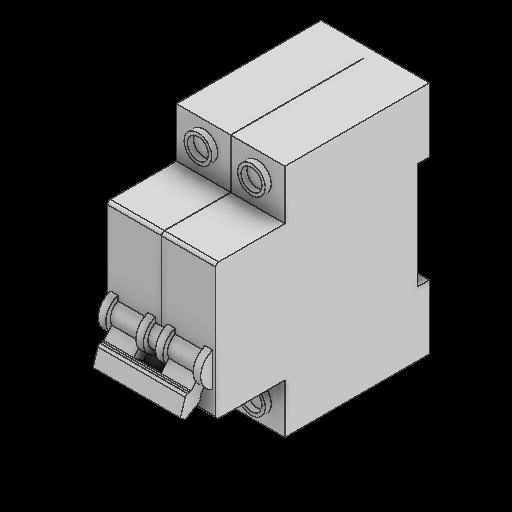
# Autodesk Inventor part: Breaker
Saved by Autodesk Inventor 2025.2 (Build 292293000, 293)
## iProperties
Created: 2026-05-14
Part Number: Breaker
Material: Generic
Document SubType Name: Modeling
Designer: valer
Density: 1 g/cm^3
Appearance: Default
Author: valer
Autodesk Inventor part; units mm, degrees
ref_plane "YZ Plane" through (0, 0, 0) normal (1, 0, 0) x (0, 1, 0)
ref_plane "XZ Plane" through (0, 0, 0) normal (0, 1, 0) x (-1, 0, 0)
ref_plane "XY Plane" through (0, 0, 0) normal (0, 0, 1) x (1, 0, 0)
sketch "Base" plane through (0, 0, 0) normal (0, 0, 1) x (1, 0, 0)
  line L0 (-18, -39) -> (18, -39)
  line L1 (18, -39) -> (18, 39)
  line L2 (18, 39) -> (-18, 39)
  line L3 (-18, 39) -> (-18, -39)
  line L4 (-18, -39) -> (18, 39) construction
  line L5 (18, -39) -> (-18, 39) construction
  point P0 (0, 0)
  dimension "d0" = 78
  dimension "d1" = 36
  constraints: 12 end point, 2 midpoint, 2 parallel, 1 horizontal, 1 perpendicular
  measures "d0" distance of L2.end L0.start
  measures "d1" distance of L0.start L0.end
extrude "BaseFeature" add sketch "Base" along normal blind 48
sketch "DINRail" plane through (-18, -39, 0) normal (-1, 0, 0) x (0, 0, 1)
  line L0 (0, 78) -> (0, 0) construction
  line L1 (0, 0) -> (48, 0) construction
  line L2 (48, 78) -> (48, 0) construction
  line L3 (0, 78) -> (48, 78) construction
  line L4 (0, 56.7) -> (4, 56.7)
  line L5 (4, 56.7) -> (4, 21.3)
  line L6 (4, 21.3) -> (0, 21.3)
  line L7 (0, 21.3) -> (0, 56.7)
  line L8 (0, 56.7) -> (4, 21.3) construction
  line L9 (4, 56.7) -> (0, 21.3) construction
  line L10 (0, -15.6) -> (0, 93.6) projected
  line L11 (-9.6, 39) -> (57.6, 39) construction
  line L12 (0, 78) -> (0, 0) projected
  point P0 (2, 39)
  dimension "d4" = 4
  dimension "d5" = 35.4
  constraints: 12 end point, 2 midpoint, 2 parallel, 1 horizontal, 1 perpendicular, 1 point on line, 1 vertical, 2 other
  measures "d4" distance of L4.start L4.end
  measures "d5" distance of L6.end L4.start
extrude "DinRailFeature" cut sketch "DINRail" against normal through all
sketch "Top" plane through (0, 0, 48) normal (0, 0, 1) x (1, 0, 0)
  line L0 (18, -39) -> (18, 39) projected
  line L1 (-18, -22.5) -> (18, -22.5)
  line L2 (18, -22.5) -> (18, 22.5)
  line L3 (18, 22.5) -> (-18, 22.5)
  line L4 (-18, 22.5) -> (-18, -22.5)
  line L5 (-18, -22.5) -> (18, 22.5) construction
  line L6 (18, -22.5) -> (-18, 22.5) construction
  point P0 (0, 0)
  point P1 (18, -22.5)
  dimension "d31" = 45
  constraints: 12 end point, 2 midpoint, 2 parallel, 1 horizontal, 1 perpendicular, 1 point on line
  measures "d31" distance between parallel lines of L1 L3
extrude "TopFeature" add sketch "Top" along normal blind 23
fillet "TopFilletsFeature" radius 1 2 edges at (0, 22.5, 71) (0, -22.5, 71)
sketch "Sketch17" plane through (0, 0, 71) normal (0, 0, 1) x (1, 0, 0)
  line L0 (18, 39) -> (-18, 39) projected
  line L1 (-18, -39) -> (18, -39) projected
  line L2 (-0.05, 39) -> (0.05, 39)
  line L3 (0.05, 39) -> (0.05, -39)
  line L4 (0.05, -39) -> (-0.05, -39)
  line L5 (-0.05, -39) -> (-0.05, 39)
  line L6 (0, -54.6) -> (0, 54.6) construction
  point P0 (0, 0)
  point P1 (0, 39)
  dimension "d71" = 0.1
  constraints: 8 end point, 3 point on line, 2 parallel, 1 horizontal, 1 midpoint, 1 perpendicular
  measures "d71" distance between parallel lines of L3 L5
sketch "SwitchHood" plane through (18, -39, 48) normal (1, 0, 0) x (0, 0, -1)
  line L0 (-23, 60.5) -> (-23, 17.5) projected
  circle A0 centre (-21, 30.5) radius 6
  line L1 (-21, 30.5) -> (-27, 30.5) construction
  line L2 (-21, 30.5) -> (-21, 24.5) construction
  line L3 (0, 16.5) -> (-22, 16.5) projected
  point P0 (48, 39)
  point P1 (-23, 24.8431)
  point P2 (-23, 36.1569)
  dimension "d35" = 12
  dimension "d36" = 4
  dimension "d37" = 8
  constraints: 4 end point, 2 point on circle, 1 centre point, 1 horizontal, 1 vertical
  measures "d35" diameter of A0
  measures "d36" distance from line of L0 L1.end
  measures "d37" distance from line of L2.end L3
extrude "SwitchHoodFeature" add sketch "SwitchHood" against normal up to surface (36 mm away) contours L0 A0 picked at (-25.1519, 30.9874)
sketch "SwithCuts" plane through (0, 0, 71) normal (0, 0, 1) x (1, 0, 0)
  line L0 (18, -2.8431) -> (18, 21.5) projected
  line L1 (18, -14.1569) -> (-18, -14.1569) projected
  line L2 (18, -2.8431) -> (17, -2.8431)
  line L3 (17, -2.8431) -> (17, -14.1569)
  line L4 (17, -14.1569) -> (18, -14.1569)
  line L5 (18, -14.1569) -> (18, -2.8431)
  line L6 (0, 54.6) -> (0, -54.6) construction
  line L7 (-18, -2.8431) -> (-17, -2.8431)
  line L8 (-17, -2.8431) -> (-17, -14.1569)
  line L9 (-17, -14.1569) -> (-18, -14.1569)
  line L10 (-18, -14.1569) -> (-18, -2.8431)
  line L11 (-18, -2.8431) -> (18, -2.8431) projected
  line L12 (-2, -2.8431) -> (2, -2.8431)
  line L13 (2, -2.8431) -> (2, -14.1569)
  line L14 (2, -14.1569) -> (-2, -14.1569)
  line L15 (-2, -14.1569) -> (-2, -2.8431)
  line L16 (-17, -2.8431) -> (-2, -14.1569) construction
  line L17 (2, -2.8431) -> (17, -14.1569) construction
  line L18 (-14.5, -14.1569) -> (-4.5, -14.1569)
  line L19 (-4.5, -14.1569) -> (-4.5, -2.8431)
  line L20 (-4.5, -2.8431) -> (-14.5, -2.8431)
  line L21 (-14.5, -2.8431) -> (-14.5, -14.1569)
  line L22 (-14.5, -14.1569) -> (-4.5, -2.8431) construction
  line L23 (-4.5, -14.1569) -> (-14.5, -2.8431) construction
  line L24 (14.5, -14.1569) -> (4.5, -14.1569)
  line L25 (4.5, -14.1569) -> (4.5, -2.8431)
  line L26 (4.5, -2.8431) -> (14.5, -2.8431)
  line L27 (14.5, -2.8431) -> (14.5, -14.1569)
  point P0 (0, 0)
  point P1 (-9.5, -8.5)
  point P2 (14.5, -14.1569)
  point P3 (-4.5, -14.1569)
  point P4 (-4.5, -2.8431)
  point P5 (2, -2.8431)
  dimension "d40" = 1
  dimension "d41" = 2
  dimension "d42" = 2
  dimension "d43" = 10
  constraints: 48 end point, 8 symmetric about line, 6 parallel, 3 horizontal, 3 midpoint, 3 perpendicular, 3 point on line, 1 collinear
  measures "d40" distance between parallel lines of L5 L3
  measures "d41" distance between parallel lines of L13 L6
  measures "d42" distance between parallel lines of L15 L6
  measures "d43" distance of L19.end L20.end
extrude "SwitchCutsFeature" cut sketch "SwithCuts" along normal through all contours L1 L3 L2 L5 | L1 L25 L11 L27 | L1 L15 L11 L13 | L1 L21 L11 L19 | L1 L10 L7 L8
sketch "SwitchBase" plane through (-17, -14.1569, 71) normal (-1, 0, 0) x (0, 0, 1)
  arc A0 (0, 0) -> (0, 11.3137) centre (-2, 5.6569) ccw projected
  circle A1 centre (-2, 5.6569) radius 4.5
  point P0 (-71, 14.1569)
  dimension "d46" = 1.5
  constraints: 1 centre point, 1 coincident
  measures "d46" radial gap between concentric circles of A0 A1
extrude "SwitchBaseFeature" add sketch "SwitchBase" against normal up to surface (34 mm away)
sketch "Sketch12" plane through (-14.5, -14.1569, 71) normal (-1, 0, 0) x (0, 0, 1)
  arc A0 (0, 1.6257) -> (0, 9.688) centre (-2, 5.6569) ccw projected
  line L0 (-9.8725, 18.5806) -> (8.9836, -4.7527)
  line L1 (8.9836, -4.7527) -> (5.8725, -7.2669)
  line L2 (5.8725, -7.2669) -> (-12.9836, 16.0664)
  line L3 (-12.9836, 16.0664) -> (-9.8725, 18.5806)
  line L4 (-9.8725, 18.5806) -> (5.8725, -7.2669) construction
  line L5 (8.9836, -4.7527) -> (-12.9836, 16.0664) construction
  point P0 (-71, 14.1569)
  point P1 (-2, 5.6569)
  point P2 (0, 0)
  dimension "d49" = 4
  dimension "d50" = 15
  constraints: 12 end point, 3 midpoint, 2 parallel, 1 perpendicular, 1 point on line
  measures "d49" distance of L0.end L1.end
  measures "d50" distance from line of point (-2, 5.657) L1
extrude "Extrusion12" add sketch "Sketch12" against normal up to surface (29 mm away)
sketch "Sketch13" plane through (-14.5, -14.1569, 71) normal (-1, 0, 0) x (0, 0, 1)
  line L0 (8.9836, -4.7527) -> (3.1111, 2.5142) projected
  line L1 (4.6442, 0.6171) -> (5.287, 0.6171)
  line L2 (5.287, 0.6171) -> (5.6013, 0.2282)
  line L3 (5.6013, 0.2282) -> (5.9902, 0.5425)
  line L4 (5.9902, 0.5425) -> (6.6187, -0.2353)
  line L5 (6.6187, -0.2353) -> (8.2059, -5.3813)
  line L6 (5.8725, -7.2669) -> (8.9836, -4.7527) projected
  arc A0 (3.1111, 2.5142) -> (0, 11.3137) centre (-2, 5.6569) ccw projected
  line L7 (7.4281, -6.0098) -> (-2, 5.6569) construction
  line L8 (1.5331, -1.8971) -> (1.3981, -2.5256)
  line L9 (1.3981, -2.5256) -> (1.7124, -2.9145)
  line L10 (1.7124, -2.9145) -> (1.3235, -3.2288)
  line L11 (1.3235, -3.2288) -> (1.9521, -4.0065)
  line L12 (1.9521, -4.0065) -> (6.6503, -6.6384)
  line L13 (0, 0) -> (5.8725, -7.2669) projected
  point P0 (-71, 14.1569)
  point P1 (4.3012, -5.3224)
  point P2 (7.4123, -2.8083)
  point P3 (6.6503, -6.6384)
  dimension "d53" = 6
  dimension "d54" = 1
  dimension "d55" = 0.5
  dimension "d56" = 0.5
  dimension "d57" = 0.5
  dimension "d58" = 1
  constraints: 22 end point, 6 symmetric about line, 2 perpendicular, 2 point on line, 1 horizontal, 1 midpoint, 1 parallel
  measures "d53" distance between parallel lines of L6 L3
  measures "d54" distance of L3.end L4.end
  measures "d55" distance of L2.end L3.end
  measures "d56" distance between parallel lines of L0 L2
  measures "d57" distance of L1.end L2.end
  measures "d58" distance of L5.end L0.start
extrude "Extrusion13" add sketch "Sketch13" against normal up to surface (29 mm away) contours L0 L1 L2 L3 L4 L5 | L12 L11 L10 L9 L8 L13
extrude "Extrusion14" cut sketch "Sketch13" against normal through all contours L6 L5 L0 | L13 L12 L6
sketch "Sketch14" plane through (4.5, -10.3782, 73.0893) normal (0, 0.6285394, 0.7777778) x (1, 0, 0)
  line L0 (-19, -4.0648) -> (10, -4.0648) projected
  line L1 (10, -4.0648) -> (10, -1.6257) projected
  line L2 (10, 0) -> (10, -1.6257) projected
  line L3 (0, 0) -> (10, 0) projected
  line L4 (0, -1.6257) -> (0, 0) projected
  line L5 (-2.5, -1.6257) -> (0, -1.6257) projected
  line L6 (-2.5, 0) -> (-2.5, -1.6257) projected
  line L7 (-6.5, 0) -> (-2.5, 0) projected
  line L8 (-6.5, -1.6257) -> (-6.5, 0) projected
  line L9 (-9, -1.6257) -> (-6.5, -1.6257) projected
  line L10 (-9, 0) -> (-9, -1.6257) projected
  line L11 (-19, 0) -> (-9, 0) projected
  line L12 (-19, -1.6257) -> (-19, 0) projected
  line L13 (-19, -4.0648) -> (-19, -1.6257) projected
  line L14 (-9, -1.6257) -> (-9, -4.0648)
  line L15 (-19, -4.0648) -> (10, -4.0648) projected
  line L16 (0, -1.6257) -> (0, -4.0648)
  point P0 (-4.5, 54.0115)
  point P1 (-9, -4.0648)
  constraints: 4 end point, 2 perpendicular, 2 point on line
extrude "Extrusion15" cut sketch "Sketch14" against normal up to surface (4 mm away) contours L14 L9 L8 L7 L6 L5 L16 L0
sketch "Sketch15" plane through (0, 0, 48) normal (0, 0, 1) x (1, 0, 0)
  line L0 (0, -54.6) -> (0, 54.6) construction
  circle A0 centre (-8.9, 31.65) radius 4.6
  line L1 (-8.9, 31.65) -> (-13.5, 31.65) construction
  line L2 (-8.9, 31.65) -> (-8.9, 36.25) construction
  line L3 (18, 39) -> (-18, 39) projected
  circle A1 centre (8.9, 31.65) radius 4.6
  line L4 (-25.2, 0) -> (25.2, 0) construction
  circle A2 centre (-8.9, -31.65) radius 4.6
  circle A3 centre (8.9, -31.65) radius 4.6
  line L5 (8.9, 31.65) -> (13.5, 31.65) construction
  line L6 (-8.9, -31.65) -> (-8.9, -36.25) construction
  circle A4 centre (-8.9, 31.65) radius 3.5
  circle A5 centre (8.9, 31.65) radius 3.5
  circle A6 centre (-8.9, -31.65) radius 3.5
  circle A7 centre (8.9, -31.65) radius 3.5
  point P0 (0, 0)
  dimension "d65" = 9.2
  dimension "d66" = 27
  dimension "d67" = 72.5
  dimension "d68" = 7
  constraints: 8 end point, 6 centre point, 4 coincident, 3 equal radius, 3 symmetric about line, 2 horizontal, 2 point on circle, 1 horizontal alignment, 1 perpendicular, 1 vertical, 1 vertical alignment, 7 other
  measures "d65" diameter of A0
  measures "d66" distance of L5.end L1.end
  measures "d67" distance of L2.end L6.end
  measures "d68" diameter of A4
extrude "Extrusion16" add sketch "Sketch15" along normal blind 2
extrude "Extrusion17" cut sketch "Sketch17" against normal up to surface (67 mm away)
body "Solid1"
